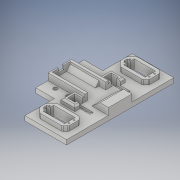
# Autodesk Inventor part: Elevator Slide
Saved by Autodesk Inventor 2018 (Build 220112000, 112)
## iProperties
Created: 2017-10-23
Part Number: Elevator Slide
Material: Generic
Document SubType Name: Modeling
Designer: thompson.nathaniel
Density: 1 g/cm^3
Appearance: Default
Author: thompson.nathaniel
Autodesk Inventor part; units mm, degrees
ref_plane "YZ Plane" through (0, 0, 0) normal (1, 0, 0) x (0, 1, 0)
ref_plane "XZ Plane" through (0, 0, 0) normal (0, 1, 0) x (-1, 0, 0)
ref_plane "XY Plane" through (0, 0, 0) normal (0, 0, 1) x (1, 0, 0)
sketch "Sketch1" plane through (0, 0, 0) normal (0, 1, 0) x (-1, 0, 0)
  line L0 (0, 0) -> (-114.3, 0)
  line L1 (-114.3, 0) -> (-114.3, 152.4)
  line L2 (-114.3, 152.4) -> (0, 152.4)
  line L3 (0, 152.4) -> (0, 0)
  line L4 (-69.85, 34.925) -> (-55.88, 34.925)
  line L5 (-55.88, 34.925) -> (-55.88, 48.895)
  line L6 (-55.88, 48.895) -> (-69.85, 48.895)
  line L7 (-69.85, 48.895) -> (-69.85, 34.925)
  line L8 (-69.85, 103.505) -> (-55.88, 103.505)
  line L9 (-55.88, 103.505) -> (-55.88, 117.475)
  line L10 (-55.88, 117.475) -> (-69.85, 117.475)
  line L11 (-69.85, 117.475) -> (-69.85, 103.505)
  dimension "d0" = 152.4
  dimension "d1" = 114.3
  dimension "d2" = 44.45
  dimension "d3" = 44.45
  dimension "d4" = 13.97
  dimension "d5" = 13.97
  dimension "d6" = 13.97
  dimension "d7" = 13.97
  dimension "d8" = 54.61
  dimension "d9" = 34.925
  constraints: 24 end point, 6 parallel, 3 horizontal, 3 perpendicular
  measures "d0" distance of L0.end L1.end
  measures "d1" distance of L0.start L0.end
  measures "d2" distance between parallel lines of L1 L7
  measures "d3" distance between parallel lines of L1 L11
  measures "d4" distance of L8.start L8.end
  measures "d5" distance of L10.end L8.start
  measures "d6" distance of L6.end L4.start
  measures "d7" distance of L4.start L4.end
  measures "d8" distance between parallel lines of L8 L6
  measures "d9" distance between parallel lines of L2 L10
extrude "Extrusion1" add sketch "Sketch1" along normal blind 10.16
sketch "Sketch2" plane through (0, 10.16, 0) normal (0, 1, 0) x (1, 0, 0)
  line L0 (49.53, -28.575) -> (76.2, -28.575)
  line L1 (76.2, -28.575) -> (76.2, -55.245)
  line L2 (76.2, -55.245) -> (49.53, -55.245)
  line L3 (49.53, -55.245) -> (49.53, -28.575)
  line L4 (49.53, -97.155) -> (76.2, -97.155)
  line L5 (76.2, -97.155) -> (76.2, -123.825)
  line L6 (76.2, -123.825) -> (49.53, -123.825)
  line L7 (49.53, -123.825) -> (49.53, -97.155)
  line L8 (55.88, -34.925) -> (69.85, -34.925) projected
  line L9 (69.85, -34.925) -> (69.85, -48.895) projected
  line L10 (69.85, -48.895) -> (55.88, -48.895) projected
  line L11 (55.88, -48.895) -> (55.88, -34.925) projected
  line L12 (55.88, -103.505) -> (69.85, -103.505) projected
  line L13 (69.85, -103.505) -> (69.85, -117.475) projected
  line L14 (69.85, -117.475) -> (55.88, -117.475) projected
  line L15 (55.88, -117.475) -> (55.88, -103.505) projected
  line L16 (55.88, -103.505) -> (55.88, -117.475)
  point P0 (0, 0)
  dimension "d12" = 6.35
  dimension "d13" = 6.35
  dimension "d14" = 6.35
  dimension "d15" = 6.35
  dimension "d16" = 6.35
  dimension "d17" = 6.35
  dimension "d18" = 6.35
  constraints: 18 end point, 5 equal length, 2 horizontal, 2 perpendicular, 1 point on line
  measures "d12" distance between parallel lines of L8 L0
  measures "d13" distance between parallel lines of L9 L1
  measures "d14" distance between parallel lines of L10 L2
  measures "d15" distance between parallel lines of L11 L3
  measures "d16" distance between parallel lines of L12 L4
  measures "d17" distance between parallel lines of L13 L5
  measures "d18" distance between parallel lines of L6 L14
extrude "Extrusion2" add sketch "Sketch2" along normal blind 8.89
chamfer "Chamfer1" distance 3.175 angle 45 8 edges at (62.865, 19.05, 123.825) (49.53, 19.05, 110.49) (62.865, 19.05, 97.155) (76.2, 19.05, 110.49) (62.865, 19.05, 55.245) (49.53, 19.05, 41.91) (62.865, 19.05, 28.575) (76.2, 19.05, 41.91)
sketch "Sketch3" plane through (0, 19.05, 0) normal (0, 1, 0) x (1, 0, 0)
  line L0 (69.85, -48.895) -> (69.85, -34.925) projected
  line L1 (76.2, -28.575) -> (76.2, -55.245) projected
  line L2 (69.85, -38.1) -> (76.2, -38.1)
  line L3 (76.2, -38.1) -> (76.2, -44.45)
  line L4 (76.2, -44.45) -> (69.85, -44.45)
  line L5 (69.85, -44.45) -> (69.85, -38.1)
  line L6 (69.85, -117.475) -> (69.85, -103.505) projected
  line L7 (76.2, -97.155) -> (76.2, -123.825) projected
  line L8 (69.85, -107.95) -> (76.2, -107.95)
  line L9 (76.2, -107.95) -> (76.2, -114.3)
  line L10 (76.2, -114.3) -> (69.85, -114.3)
  line L11 (69.85, -114.3) -> (69.85, -107.95)
  line L12 (55.88, -34.925) -> (69.85, -34.925) projected
  line L13 (69.85, -117.475) -> (55.88, -117.475) projected
  point P0 (0, 0)
  dimension "d24" = 6.35
  dimension "d25" = 3.175
  dimension "d26" = 3.175
  dimension "d27" = 6.35
  constraints: 16 end point, 4 parallel, 4 point on line, 2 horizontal, 2 perpendicular
  measures "d24" distance between parallel lines of L4 L2
  measures "d25" distance between parallel lines of L12 L2
  measures "d26" distance between parallel lines of L13 L10
  measures "d27" distance of L10.end L8.start
extrude "Extrusion3" cut sketch "Sketch3" against normal blind 8.89
sketch "Sketch4" plane through (0, 10.16, 0) normal (0, 1, 0) x (1, 0, 0)
  line L0 (69.85, -38.1) -> (95.25, -38.1)
  line L1 (95.25, -38.1) -> (95.25, -44.45)
  line L2 (95.25, -44.45) -> (69.85, -44.45)
  line L3 (69.85, -44.45) -> (69.85, -38.1)
  line L4 (69.85, -114.3) -> (69.85, -107.95) projected
  line L5 (69.85, -107.95) -> (95.25, -107.95)
  line L6 (95.25, -107.95) -> (95.25, -114.3)
  line L7 (95.25, -114.3) -> (69.85, -114.3)
  line L8 (69.85, -114.3) -> (69.85, -107.95)
  point P0 (0, 0)
  dimension "d30" = 25.4
  dimension "d31" = 6.35
  dimension "d32" = 6.35
  dimension "d33" = 25.4
  constraints: 16 end point, 4 parallel, 2 horizontal, 2 perpendicular
  measures "d30" distance of L6.end L7.end
  measures "d31" distance between parallel lines of L5 L7
  measures "d32" distance between parallel lines of L0 L2
  measures "d33" distance between parallel lines of L3 L1
extrude "Extrusion4" cut sketch "Sketch4" against normal blind 3.81
fillet "Fillet1" radius 21.336 2 edges at (95.25, 6.35, 41.275) (95.25, 6.35, 111.125)
sketch "Sketch5" plane through (0, 10.16, 0) normal (0, 1, 0) x (1, 0, 0)
  line L0 (0, -152.4) -> (0, 0) projected
  line L1 (0, -98.425) -> (100.33, -98.425)
  line L2 (100.33, -98.425) -> (100.33, -53.975)
  line L3 (100.33, -53.975) -> (0, -53.975)
  line L4 (0, -53.975) -> (0, -98.425)
  line L5 (49.53, -97.155) -> (76.2, -97.155) projected
  dimension "d37" = 44.45
  dimension "d38" = 1.27
  dimension "d39" = 100.33
  constraints: 8 end point, 2 parallel, 1 horizontal, 1 perpendicular, 1 point on line
  measures "d37" distance between parallel lines of L3 L1
  measures "d38" distance between parallel lines of L5 L1
  measures "d39" distance between parallel lines of L0 L2
extrude "Extrusion5" add sketch "Sketch5" along normal blind 12.7
sketch "Sketch6" plane through (100.33, 10.16, 98.425) normal (1, 0, 0) x (0, 0, -1)
  line L0 (44.45, 12.7) -> (0, 12.7) projected
  line L1 (5.08, 12.7) -> (5.08, 8.89)
  line L2 (5.08, 8.89) -> (11.811, 0)
  line L3 (44.45, 0) -> (0, 0) projected
  line L4 (32.639, 0) -> (39.37, 8.89)
  line L5 (39.37, 8.89) -> (39.37, 12.7)
  line L6 (5.08, 12.7) -> (39.37, 12.7)
  line L7 (0, 12.7) -> (44.45, 12.7) projected
  line L8 (0, 0) -> (0, 12.7) projected
  point P0 (98.425, -10.16)
  dimension "d42" = 34.29
  dimension "d43" = 5.08
  dimension "d44" = 20.828
  dimension "d45" = 8.89
  dimension "d46" = 8.89
  dimension "d47" = 6.731
  constraints: 10 end point, 4 point on line, 1 collinear, 1 parallel, 1 vertical
  measures "d42" distance between parallel lines of L5 L1
  measures "d43" distance between parallel lines of L8 L1
  measures "d44" distance of L4.start L2.end
  measures "d45" distance from line of L3 L1.end
  measures "d46" distance from line of L3 L4.end
  measures "d47" distance from line of L1 L2.end
extrude "Extrusion6" cut sketch "Sketch6" against normal blind 100.33 contours L5 L4 L3 L2 L1 L0
sketch "Sketch7" plane through (0, 22.86, 0) normal (0, 1, 0) x (1, 0, 0)
  line L0 (0, -98.425) -> (100.33, -98.425) projected
  line L1 (76.2, -53.975) -> (100.33, -53.975) projected
  line L2 (100.33, -98.425) -> (96.52, -98.425)
  line L3 (96.52, -98.425) -> (96.52, -53.975)
  line L4 (96.52, -53.975) -> (100.33, -53.975)
  line L5 (100.33, -53.975) -> (100.33, -98.425)
  point P0 (0, 0)
  dimension "d50" = 3.81
  constraints: 8 end point, 2 parallel, 1 horizontal, 1 perpendicular, 1 point on line
  measures "d50" distance between parallel lines of L5 L3
extrude "Extrusion7" add sketch "Sketch7" against normal blind 12.7
sketch "Sketch8" plane through (0, 22.86, 0) normal (0, 1, 0) x (1, 0, 0)
  line L0 (100.33, -98.425) -> (76.2, -98.425) projected
  line L1 (76.2, -53.975) -> (100.33, -53.975) projected
  line L2 (76.2, -98.425) -> (96.52, -98.425)
  line L3 (96.52, -98.425) -> (96.52, -53.975)
  line L4 (96.52, -53.975) -> (76.2, -53.975)
  line L5 (76.2, -53.975) -> (76.2, -98.425)
  point P0 (0, 0)
  constraints: 8 end point, 2 parallel, 1 horizontal, 1 perpendicular, 1 point on line
extrude "Extrusion8" cut sketch "Sketch8" against normal blind 12.7
sketch "Sketch9" plane through (100.33, 10.16, 98.425) normal (1, 0, 0) x (0, 0, -1)
  line L0 (0, 12.7) -> (44.45, 12.7) projected
  line L1 (44.45, 0) -> (0, 0) projected
  line L2 (0, 12.7) -> (44.45, 12.7)
  line L3 (44.45, 12.7) -> (44.45, 0)
  line L4 (44.45, 0) -> (0, 0)
  line L5 (0, 0) -> (0, 12.7)
  point P0 (98.425, -10.16)
  constraints: 8 end point, 2 parallel, 1 horizontal, 1 perpendicular
extrude "Extrusion9" add sketch "Sketch9" along normal blind 6.35
sketch "Sketch10" plane through (106.68, 10.16, 98.425) normal (1, 0, 0) x (0, 0, -1)
  line L0 (44.45, 0) -> (44.45, 12.7) projected
  line L1 (-25.4, 0) -> (0, 0) projected
  line L2 (44.45, 12.7) -> (0, 12.7)
  line L3 (0, 12.7) -> (0, 0)
  line L4 (0, 0) -> (44.45, 0)
  line L5 (44.45, 0) -> (44.45, 12.7)
  point P0 (98.425, -10.16)
  constraints: 8 end point, 2 parallel, 1 horizontal, 1 perpendicular
extrude "Extrusion10" add sketch "Sketch10" along normal blind 7.62
sketch "Sketch11" plane through (96.52, 22.86, 53.975) normal (-1, 0, 0) x (0, 0, 1)
  line L0 (0, -12.7) -> (0, 0) projected
  line L1 (44.45, 0) -> (44.45, -12.7) projected
  line L2 (0, -12.7) -> (44.45, -12.7)
  line L3 (44.45, -12.7) -> (44.45, 0)
  line L4 (44.45, 0) -> (0, 0)
  line L5 (0, 0) -> (0, -12.7)
  point P0 (-53.975, -22.86)
  constraints: 8 end point, 2 parallel, 1 horizontal, 1 perpendicular
extrude "Extrusion11" cut sketch "Sketch11" against normal blind 5.08
sketch "Sketch12" plane through (0, 22.86, 0) normal (0, 1, 0) x (1, 0, 0)
  line L0 (76.2, -59.055) -> (76.2, -53.975) projected
  line L1 (76.2, -93.345) -> (0, -93.345) projected
  line L2 (76.2, -59.055) -> (57.15, -59.055)
  line L3 (57.15, -59.055) -> (57.15, -93.345)
  line L4 (57.15, -93.345) -> (76.2, -93.345)
  line L5 (76.2, -93.345) -> (76.2, -59.055)
  line L6 (0, -93.345) -> (0, -98.425) projected
  point P0 (0, 0)
  dimension "d61" = 57.15
  constraints: 8 end point, 2 parallel, 1 horizontal, 1 perpendicular, 1 point on line
  measures "d61" distance between parallel lines of L6 L3
extrude "Extrusion12" cut sketch "Sketch12" against normal blind 12.7
sketch "Sketch13" plane through (101.6, 22.86, 53.975) normal (-1, 0, 0) x (0, 0, 1)
  line L0 (0, -12.7) -> (44.45, -12.7)
  line L1 (44.45, -12.7) -> (44.45, 0)
  line L2 (44.45, 0) -> (0, 0)
  line L3 (0, 0) -> (0, -12.7)
  point P0 (-53.975, -22.86)
  constraints: 8 end point, 2 parallel, 1 horizontal, 1 perpendicular
extrude "Extrusion13" cut sketch "Sketch13" along normal blind 31.75
sketch "Sketch14" plane through (69.85, 19.05, 107.95) normal (0, 0, 1) x (1, 0, 0)
  line L0 (6.35, -8.89) -> (25.4, -8.89) projected
  line L1 (0, 0) -> (6.35, 0)
  line L2 (6.35, 0) -> (6.35, -8.89)
  line L3 (6.35, -8.89) -> (0, -8.89)
  line L4 (0, -8.89) -> (0, 0)
  point P0 (-69.85, -19.05)
  dimension "d66" = 6.35
  dimension "d67" = 8.89
  constraints: 8 end point, 2 parallel, 1 horizontal, 1 perpendicular
  measures "d66" distance of L1.start L1.end
  measures "d67" distance of L1.end L0.start
extrude "Extrusion14" cut sketch "Sketch14" against normal blind 63.5
sketch "Sketch15" plane through (0, 10.16, 0) normal (0, 1, 0) x (1, 0, 0)
  circle A0 centre (20.32, -104.775) radius 3.81
  circle A1 centre (44.45, -104.775) radius 3.81
  circle A2 centre (20.32, -47.625) radius 3.81
  circle A3 centre (44.45, -47.625) radius 3.81
  line L0 (0, -98.425) -> (0, -152.4) projected
  line L1 (0, -53.975) -> (49.53, -53.975) projected
  line L2 (0, 0) -> (0, -53.975) projected
  line L3 (49.53, -98.425) -> (0, -98.425) projected
  dimension "d70" = 7.62
  dimension "d71" = 7.62
  dimension "d72" = 7.62
  dimension "d73" = 7.62
  dimension "d74" = 20.32
  dimension "d75" = 44.45
  dimension "d76" = 6.35
  dimension "d77" = 20.32
  dimension "d78" = 44.45
  dimension "d79" = 6.35
  dimension "d80" = 6.35
  dimension "d81" = 6.35
  constraints: 4 centre point
  measures "d70" diameter of A0
  measures "d71" diameter of A2
  measures "d72" diameter of A3
  measures "d73" diameter of A1
  measures "d74" distance from line of L0 A0.centre
  measures "d75" distance from line of L0 A1.centre
  measures "d76" distance from line of L1 A3.centre
  measures "d77" distance from line of L2 A2.centre
  measures "d78" distance from line of L2 A3.centre
  measures "d79" distance from line of L1 A2.centre
  measures "d80" distance from line of L3 A0.centre
  measures "d81" distance from line of L3 A1.centre
extrude "Extrusion15" cut sketch "Sketch15" against normal blind 10.16
sketch "Sketch16" plane through (0, 0, 152.4) normal (0, 0, 1) x (1, 0, 0)
  line L0 (57.15, 10.16) -> (0, 10.16) projected
  line L1 (114.3, 0) -> (0, 0) projected
  line L2 (0, 10.16) -> (114.3, 10.16)
  line L3 (114.3, 10.16) -> (114.3, 0)
  line L4 (114.3, 0) -> (0, 0)
  line L5 (0, 0) -> (0, 10.16)
  constraints: 8 end point, 2 parallel, 1 horizontal, 1 perpendicular
extrude "Extrusion16" add sketch "Sketch16" along normal blind 25.4
sketch "Sketch17" plane through (114.3, 0, 0) normal (0, 0, -1) x (-1, 0, 0)
  line L0 (114.3, 10.16) -> (114.3, 19.05) projected
  line L1 (0, 0) -> (0, 10.16) projected
  line L2 (114.3, 10.16) -> (0, 10.16)
  line L3 (0, 10.16) -> (0, 0)
  line L4 (0, 0) -> (114.3, 0)
  line L5 (114.3, 0) -> (114.3, 10.16)
  constraints: 8 end point, 2 parallel, 1 horizontal, 1 perpendicular
extrude "Extrusion17" add sketch "Sketch17" along normal blind 25.4
sketch "Sketch18" plane through (0, 0, 0) normal (0, -1, 0) x (1, 0, 0)
  line L0 (114.3, -25.4) -> (0, -25.4) projected
  line L1 (114.3, -25.4) -> (0, -25.4)
  line L2 (0, -25.4) -> (0, 177.8)
  line L3 (0, 177.8) -> (114.3, 177.8)
  line L4 (114.3, 177.8) -> (114.3, -25.4)
  line L5 (0, 177.8) -> (114.3, 177.8) projected
  point P0 (0, 0)
  dimension "d88" = 0
  dimension "d89" = 114.3
  constraints: 8 end point, 2 parallel, 1 horizontal, 1 perpendicular
  measures "d88" distance between parallel lines of L5 L3
  measures "d89" distance between parallel lines of L2 L4
extrude "Extrusion18" cut sketch "Sketch18" against normal blind 1.27
sketch "Sketch25" plane through (101.6, 22.86, 53.975) normal (-1, 0, 0) x (0, 0, 1)
  line L0 (0, -12.7) -> (0, 0) projected
  line L1 (0, 0) -> (44.45, 0) projected
  line L2 (0, -12.7) -> (44.45, -12.7)
  line L3 (44.45, -12.7) -> (44.45, 0)
  line L4 (44.45, 0) -> (0, 0)
  line L5 (0, 0) -> (0, -12.7)
  point P0 (-53.975, -22.86)
  constraints: 8 end point, 2 parallel, 1 horizontal, 1 perpendicular
extrude "Extrusion25" add sketch "Sketch25" along normal blind 3.0734
sketch "Sketch26" plane through (0, 10.16, 0) normal (0, 1, 0) x (1, 0, 0)
  line L0 (98.5266, -53.975) -> (83.2866, -53.975)
  line L1 (83.2866, -53.975) -> (83.2866, -98.425)
  line L2 (83.2866, -98.425) -> (98.5266, -98.425)
  line L3 (98.5266, -98.425) -> (98.5266, -53.975)
  line L4 (114.3, -98.425) -> (98.5266, -98.425) projected
  point P0 (0, 0)
  dimension "d140" = 0
  dimension "d141" = 15.24
  constraints: 8 end point, 2 parallel, 1 horizontal, 1 perpendicular
  measures "d140" distance between parallel lines of L4 L2
  measures "d141" distance between parallel lines of L3 L1
extrude "Extrusion26" add sketch "Sketch26" along normal blind 12.954
chamfer "Chamfer4" distance 15.24 distance2 12.954 1 edges at (83.2866, 23.114, 76.2) measured on face at (93.4466, 23.114, 83.6083)
sketch "Sketch27" plane through (0, 22.86, 0) normal (0, 1, 0) x (1, 0, 0)
  line L0 (98.5266, -98.425) -> (98.5266, -53.975) projected
  line L1 (98.5266, -53.975) -> (114.3, -53.975) projected
  line L2 (98.5266, -98.425) -> (114.3, -98.425)
  line L3 (114.3, -98.425) -> (114.3, -53.975)
  line L4 (114.3, -53.975) -> (98.5266, -53.975)
  line L5 (98.5266, -53.975) -> (98.5266, -98.425)
  point P0 (0, 0)
  constraints: 8 end point, 2 parallel, 1 horizontal, 1 perpendicular
extrude "Extrusion27" add sketch "Sketch27" along normal blind 0.254
sketch "Sketch28" plane through (0, 22.86, 0) normal (0, 1, 0) x (1, 0, 0)
  line L0 (0, -93.345) -> (0, -98.425) projected
  line L1 (69.85, -53.975) -> (0, -53.975) projected
  line L2 (0, -98.425) -> (2.54, -98.425)
  line L3 (2.54, -98.425) -> (2.54, -53.975)
  line L4 (2.54, -53.975) -> (0, -53.975)
  line L5 (0, -53.975) -> (0, -98.425)
  point P0 (0, 0)
  dimension "d149" = 2.54
  constraints: 8 end point, 2 parallel, 1 horizontal, 1 perpendicular, 1 point on line
  measures "d149" distance between parallel lines of L5 L3
extrude "Extrusion28" add sketch "Sketch28" against normal blind 12.7
sketch "Sketch29" plane through (2.54, 22.86, 93.345) normal (1, 0, 0) x (0, 0, -1)
  line L0 (12.065, -6.858) -> (22.225, -6.858)
  line L1 (22.225, -6.858) -> (22.225, 0)
  line L2 (22.225, 0) -> (12.065, 0)
  line L3 (12.065, 0) -> (12.065, -6.858)
  line L4 (27.559, -12.7) -> (6.731, -12.7) projected
  line L5 (0, 0) -> (34.29, 0) projected
  point P0 (93.345, -22.86)
  dimension "d152" = 5.842
  dimension "d153" = 5.334
  dimension "d154" = 5.334
  dimension "d155" = 0
  constraints: 8 end point, 2 parallel, 1 horizontal, 1 perpendicular
  measures "d152" distance between parallel lines of L4 L0
  measures "d153" distance from line of L4.start L1
  measures "d154" distance from line of L4.end L3
  measures "d155" distance between parallel lines of L2 L5
extrude "Extrusion29" cut sketch "Sketch29" against normal blind 12.7
sketch "Sketch30" plane through (0, 10.16, 0) normal (0, 1, 0) x (1, 0, 0)
  line L0 (54.61, -162.3187) -> (95.25, -162.3187)
  line L1 (95.25, -162.3187) -> (95.25, -142.4813)
  line L2 (95.25, -142.4813) -> (54.61, -142.4813)
  line L3 (54.61, -142.4813) -> (54.61, -162.3187)
  line L4 (54.61, -9.9187) -> (95.25, -9.9187)
  line L5 (95.25, -9.9187) -> (95.25, 9.9187)
  line L6 (95.25, 9.9187) -> (54.61, 9.9187)
  line L7 (54.61, 9.9187) -> (54.61, -9.9187)
  line L8 (114.3, -177.8) -> (0, -177.8) projected
  line L9 (114.3, -98.425) -> (114.3, -177.8) projected
  line L10 (114.3, -53.975) -> (114.3, 25.4) projected
  line L11 (0, 25.4) -> (114.3, 25.4) projected
  line L12 (0, -177.8) -> (35.56, -177.8)
  line L13 (35.56, -177.8) -> (35.56, -121.92)
  line L14 (35.56, -121.92) -> (0, -121.92)
  line L15 (0, -121.92) -> (0, -177.8)
  line L16 (0, 25.4) -> (0, -177.8) projected
  line L17 (0, 25.4) -> (35.56, 25.4)
  line L18 (35.56, 25.4) -> (35.56, -30.48)
  line L19 (35.56, -30.48) -> (0, -30.48)
  line L20 (0, -30.48) -> (0, 25.4)
  point P0 (0, 0)
  dimension "d158" = 19.8374
  dimension "d159" = 19.8374
  dimension "d160" = 40.64
  dimension "d161" = 40.64
  dimension "d162" = 15.4813
  dimension "d163" = 19.05
  dimension "d164" = 19.05
  dimension "d165" = 15.4813
  dimension "d168" = 55.88
  dimension "d169" = 55.88
  dimension "d170" = 35.56
  constraints: 32 end point, 8 parallel, 4 horizontal, 4 perpendicular, 1 point on line
  measures "d158" distance of L2.end L0.start
  measures "d159" distance of L6.end L4.start
  measures "d160" distance of L1.end L2.end
  measures "d161" distance of L5.end L6.end
  measures "d162" distance between parallel lines of L8 L0
  measures "d163" distance between parallel lines of L9 L1
  measures "d164" distance between parallel lines of L10 L5
  measures "d165" distance between parallel lines of L11 L6
  measures "d168" distance of L12.end L13.end
  measures "d169" distance of L17.end L18.end
  measures "d170" distance of L13.end L14.end
extrude "Extrusion31" cut sketch "Sketch30" against normal blind 25.4
sketch "Sketch31" plane through (0, 10.16, 0) normal (0, 1, 0) x (1, 0, 0)
  line L0 (46.99, -168.4147) -> (102.87, -168.4147)
  line L1 (102.87, -168.4147) -> (102.87, -136.3853)
  line L2 (102.87, -136.3853) -> (46.99, -136.3853)
  line L3 (46.99, -136.3853) -> (46.99, -168.4147)
  line L4 (54.61, -162.3187) -> (54.61, -142.4813) projected
  line L5 (95.25, -142.4813) -> (54.61, -142.4813) projected
  line L6 (54.61, -162.3187) -> (95.25, -162.3187)
  line L7 (95.25, -162.3187) -> (95.25, -142.4813)
  line L8 (95.25, -142.4813) -> (54.61, -142.4813)
  line L9 (54.61, -142.4813) -> (54.61, -162.3187)
  line L10 (95.25, -9.9187) -> (54.61, -9.9187) projected
  line L11 (95.25, 9.9187) -> (95.25, -9.9187) projected
  line L12 (54.61, -9.9187) -> (95.25, -9.9187)
  line L13 (95.25, -9.9187) -> (95.25, 9.9187)
  line L14 (95.25, 9.9187) -> (54.61, 9.9187)
  line L15 (54.61, 9.9187) -> (54.61, -9.9187)
  line L16 (46.99, -16.0147) -> (102.87, -16.0147)
  line L17 (102.87, -16.0147) -> (102.87, 16.0147)
  line L18 (102.87, 16.0147) -> (46.99, 16.0147)
  line L19 (46.99, 16.0147) -> (46.99, -16.0147)
  point P0 (0, 0)
  dimension "d173" = 7.62
  dimension "d174" = 6.096
  dimension "d175" = 6.096
  dimension "d176" = 7.62
  dimension "d177" = 6.096
  dimension "d178" = 6.096
  dimension "d179" = 7.62
  constraints: 32 end point, 8 parallel, 4 horizontal, 4 perpendicular, 1 point on line
  measures "d173" distance between parallel lines of L3 L4
  measures "d174" distance between parallel lines of L2 L5
  measures "d175" distance between parallel lines of L6 L0
  measures "d176" distance between parallel lines of L1 L7
  measures "d177" distance between parallel lines of L18 L14
  measures "d178" distance between parallel lines of L16 L10
  measures "d179" distance between parallel lines of L17 L11
extrude "Extrusion32" add sketch "Sketch31" along normal blind 8.89
sketch "Sketch32" plane through (0, 19.05, 0) normal (0, 1, 0) x (1, 0, 0)
  circle A0 centre (51.562, -157.353) radius 1.27
  circle A1 centre (51.562, -147.447) radius 1.27
  circle A2 centre (98.298, -147.447) radius 1.27
  circle A3 centre (98.298, -157.353) radius 1.27
  line L0 (46.99, -136.3853) -> (46.99, -168.4147) projected
  line L1 (102.87, -168.4147) -> (102.87, -136.3853) projected
  line L2 (102.87, -136.3853) -> (46.99, -136.3853) projected
  circle A4 centre (51.562, -4.953) radius 1.27
  circle A5 centre (51.562, 4.953) radius 1.27
  circle A6 centre (98.298, 4.953) radius 1.27
  circle A7 centre (98.298, -4.953) radius 1.27
  line L3 (46.99, 16.0147) -> (46.99, -16.0147) projected
  line L4 (102.87, -16.0147) -> (102.87, 16.0147) projected
  line L5 (46.99, -16.0147) -> (102.87, -16.0147) projected
  point P0 (0, 0)
  dimension "d185" = 4.572
  dimension "d186" = 4.572
  dimension "d187" = 4.572
  dimension "d188" = 4.572
  dimension "d189" = 9.906
  dimension "d190" = 9.906
  dimension "d191" = 11.0617
  dimension "d192" = 11.0617
  dimension "d193" = 2.54
  dimension "d194" = 2.54
  dimension "d195" = 2.54
  dimension "d196" = 2.54
  dimension "d199" = 4.572
  dimension "d200" = 4.572
  dimension "d201" = 4.572
  dimension "d202" = 4.572
  dimension "d203" = 2.54
  dimension "d204" = 2.54
  dimension "d205" = 2.54
  dimension "d206" = 2.54
  dimension "d207" = 9.906
  dimension "d208" = 9.906
  dimension "d209" = 11.0617
  dimension "d210" = 11.0617
  constraints: 8 centre point
  measures "d185" distance from line of L0 A0.centre
  measures "d186" distance from line of L0 A1.centre
  measures "d187" distance from line of L1 A2.centre
  measures "d188" distance from line of L1 A3.centre
  measures "d189" distance of A2.centre A3.centre
  measures "d190" distance of A0.centre A1.centre
  measures "d191" distance from line of L2 A2.centre
  measures "d192" distance from line of L2 A1.centre
  measures "d193" diameter of A0
  measures "d194" diameter of A1
  measures "d195" diameter of A3
  measures "d196" diameter of A2
  measures "d199" distance from line of L3 A4.centre
  measures "d200" distance from line of L3 A5.centre
  measures "d201" distance from line of L4 A6.centre
  measures "d202" distance from line of L4 A7.centre
  measures "d203" diameter of A7
  measures "d204" diameter of A6
  measures "d205" diameter of A5
  measures "d206" diameter of A4
  measures "d207" distance of A5.centre A4.centre
  measures "d208" distance of A6.centre A7.centre
  measures "d209" distance from line of L5 A7.centre
  measures "d210" distance from line of L5 A4.centre
extrude "Extrusion35" cut sketch "Sketch32" against normal blind 6.35
sketch "Sketch33" plane through (0, 19.05, 0) normal (0, 1, 0) x (1, 0, 0)
  line L0 (54.61, -162.3187) -> (54.61, -142.4813) projected
  line L1 (54.61, -155.575) -> (48.26, -155.575)
  line L2 (48.26, -155.575) -> (48.26, -149.225)
  line L3 (48.26, -149.225) -> (54.61, -149.225)
  line L4 (54.61, -149.225) -> (54.61, -155.575)
  line L5 (95.25, -142.4813) -> (95.25, -162.3187) projected
  line L6 (54.61, -3.175) -> (48.26, -3.175)
  line L7 (48.26, -3.175) -> (48.26, 3.175)
  line L8 (48.26, 3.175) -> (54.61, 3.175)
  line L9 (54.61, 3.175) -> (54.61, -3.175)
  line L10 (46.99, -136.3853) -> (46.99, -168.4147) projected
  line L11 (102.87, -168.4147) -> (102.87, -136.3853) projected
  line L12 (46.99, 16.0147) -> (46.99, -16.0147) projected
  line L13 (102.87, 16.0147) -> (46.99, 16.0147) projected
  line L14 (102.87, -136.3853) -> (46.99, -136.3853) projected
  point P0 (0, 0)
  dimension "d215" = 1.27
  dimension "d217" = 6.35
  dimension "d218" = 1.27
  dimension "d219" = 6.35
  dimension "d220" = 12.8397
  dimension "d221" = 12.8397
  constraints: 16 end point, 4 parallel, 2 horizontal, 2 perpendicular, 2 point on line
  measures "d215" distance between parallel lines of L10 L2
  measures "d217" distance of L6.end L7.end
  measures "d218" distance between parallel lines of L12 L7
  measures "d219" distance between parallel lines of L1 L3
  measures "d220" distance between parallel lines of L13 L8
  measures "d221" distance between parallel lines of L14 L3
extrude "Extrusion36" cut sketch "Sketch33" against normal blind 25.4
sketch "Sketch34" plane through (46.99, 10.16, 136.3853) normal (-1, 0, 0) x (0, 0, 1)
  line L0 (-152.4, 8.89) -> (-120.3706, 8.89) projected
  line L1 (-120.3706, 0) -> (-152.4, 0) projected
  line L2 (-152.4, 8.89) -> (-120.3706, 8.89)
  line L3 (-120.3706, 8.89) -> (-120.3706, 0)
  line L4 (-120.3706, 0) -> (-152.4, 0)
  line L5 (-152.4, 0) -> (-152.4, 8.89)
  line L6 (0, 8.89) -> (32.0294, 8.89) projected
  line L7 (0, 0) -> (0, 8.89) projected
  line L8 (32.0294, 8.89) -> (0, 8.89)
  line L9 (0, 8.89) -> (0, 0)
  line L10 (0, 0) -> (32.0294, 0)
  line L11 (32.0294, 0) -> (32.0294, 8.89)
  point P0 (-136.3853, -10.16)
  constraints: 16 end point, 4 parallel, 2 horizontal, 2 perpendicular
extrude "Extrusion37" add sketch "Sketch34" along normal blind 2.54
chamfer "Chamfer6" distance 6.35 angle 45 4 edges at (102.87, 14.605, -16.0147) (102.87, 14.605, 16.0147) (102.87, 14.605, 136.3853) (102.87, 14.605, 168.4147)
chamfer "Chamfer7" distance 10.16 angle 45 4 edges at (44.45, 14.605, 136.3853) (44.45, 14.605, 168.4147) (44.45, 14.605, 16.0147) (44.45, 14.605, -16.0147)
fillet "Fillet2" radius 3.175 16 edges at (54.61, 14.605, 16.0147) (44.45, 14.605, 5.8547) (44.45, 14.605, -5.8547) (54.61, 14.605, -16.0147) (96.52, 14.605, -16.0147) (102.87, 14.605, -9.6647) (96.52, 14.605, 16.0147) (102.87, 14.605, 9.6647) (102.87, 14.605, 162.0647) (96.52, 14.605, 168.4147) (102.87, 14.605, 142.7353) (96.52, 14.605, 136.3853) (54.61, 14.605, 168.4147) (44.45, 14.605, 158.2547) (44.45, 14.605, 146.5453) (54.61, 14.605, 136.3853)
body "Solid1"
